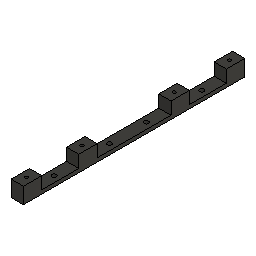
raspi_cover_holder (Autodesk Fusion 360 design; units mm, degrees)
Autodesk Fusion 360 part; units mm, degrees
sketch "Skizze1" plane through (0, 0, 0) normal (0, 0, 1) x (1, 0, 0)
  line L0 (0, 118.8766) -> (0, -120.4869) construction
  line L1 (5, -90) -> (-5, -90)
  line L2 (-5, -90) -> (-5, 90)
  line L3 (-5, 90) -> (5, 90)
  line L4 (5, 90) -> (5, -90)
  line L5 (5, -90) -> (-5, 90) construction
  line L6 (-5, -90) -> (5, 90) construction
  circle A0 centre (0, 37.5) radius 1.25
  circle A1 centre (0, -37.5) radius 1.25
  circle A2 centre (0, 15) radius 1.75
  circle A3 centre (0, -15) radius 1.75
  circle A4 centre (0, 60) radius 1.75
  circle A5 centre (0, -60) radius 1.75
  line L7 (-5, 30) -> (5, 30)
  line L8 (-5, -30) -> (5, -30)
  line L9 (-5, -45) -> (5, -45)
  line L10 (-5, 45) -> (5, 45)
  line L11 (1.2702, -39.7) -> (2.5403, -37.5)
  line L12 (2.5403, -37.5) -> (1.2702, -35.3)
  line L13 (1.2702, -35.3) -> (-1.2702, -35.3)
  line L14 (-1.2702, -35.3) -> (-2.5403, -37.5)
  line L15 (-2.5403, -37.5) -> (-1.2702, -39.7)
  line L16 (-1.2702, -39.7) -> (1.2702, -39.7)
  line L17 (1.2702, 35.3) -> (2.5403, 37.5)
  line L18 (2.5403, 37.5) -> (1.2702, 39.7)
  line L19 (1.2702, 39.7) -> (-1.2702, 39.7)
  line L20 (-1.2702, 39.7) -> (-2.5403, 37.5)
  line L21 (-2.5403, 37.5) -> (-1.2702, 35.3)
  line L22 (-1.2702, 35.3) -> (1.2702, 35.3)
  circle A6 centre (0, 82.5) radius 1.25
  circle A7 centre (0, -82.5) radius 1.25
  line L23 (1.2702, 80.3) -> (2.5403, 82.5)
  line L24 (2.5403, 82.5) -> (1.2702, 84.7)
  line L25 (1.2702, 84.7) -> (-1.2702, 84.7)
  line L26 (-1.2702, 84.7) -> (-2.5403, 82.5)
  line L27 (-2.5403, 82.5) -> (-1.2702, 80.3)
  line L28 (-1.2702, 80.3) -> (1.2702, 80.3)
  line L29 (1.2702, -84.7) -> (2.5403, -82.5)
  line L30 (2.5403, -82.5) -> (1.2702, -80.3)
  line L31 (1.2702, -80.3) -> (-1.2702, -80.3)
  line L32 (-1.2702, -80.3) -> (-2.5403, -82.5)
  line L33 (-2.5403, -82.5) -> (-1.2702, -84.7)
  line L34 (-1.2702, -84.7) -> (1.2702, -84.7)
  line L35 (-5, -75) -> (5, -75)
  line L36 (-5, 75) -> (5, 75)
  point P0 (0, -37.5)
  point P1 (0, 37.5)
  point P2 (0, 82.5)
  point P3 (0, -82.5)
  dimension "d1" = 10
  dimension "d2" = 180
  dimension "d3" = 37.5
  dimension "d4" = 37.5
  dimension "d5" = 2.5
  dimension "d7" = 2.5
  dimension "d8" = 3.5
  dimension "d9" = 3.5
  dimension "d10" = 15
  dimension "d11" = 15
  dimension "d12" = 3.5
  dimension "d13" = 3.5
  dimension "d14" = 45
  dimension "d15" = 45
  dimension "d16" = 7.5
  dimension "d17" = 7.5
  dimension "d20" = 4.4
  dimension "d21" = 4.4
  dimension "d33" = 2.5
  dimension "d34" = 2.5
  dimension "d35" = 4.4
  dimension "d36" = 4.4
  dimension "d37" = 45
  dimension "d38" = 45
  dimension "d39" = 7.5
  dimension "d40" = 7.5
  dimension "d41" = 7.5
  dimension "d42" = 7.5
  dimension "d43" = 7.5
  constraint vertical L0
  constraint coincident origin L0
  constraint horizontal L1
  constraint perpendicular L1 L2
  constraint parallel L1 L3
  constraint parallel L2 L4
  constraint coincident L5 origin
  constraint coincident L6 origin
  constraint coincident L0 P1
  constraint coincident L0 P0
  constraint coincident L0 A2.centre
  constraint coincident L0 A3.centre
  constraint coincident L0 A4.centre
  constraint coincident L0 A5.centre
  constraint coincident L2 L7.start
  constraint coincident L4 L7.end
  constraint perpendicular L4 L7
  constraint coincident L2 L8.start
  constraint coincident L4 L8.end
  constraint perpendicular L4 L8
  constraint coincident L2 L9.start
  constraint coincident L4 L9.end
  constraint perpendicular L4 L9
  constraint coincident L2 L10.start
  constraint coincident L4 L10.end
  constraint perpendicular L4 L10
  constraint coincident P0 A1.centre
  constraint coincident P1 A0.centre
  constraint horizontal L22
  constraint horizontal L16
  constraint coincident L0 P2
  constraint coincident L0 P3
  constraint coincident P2 A6.centre
  constraint coincident P3 A7.centre
  constraint horizontal L34
  constraint horizontal L28
  constraint coincident L2 L35.start
  constraint coincident L4 L35.end
  constraint perpendicular L4 L35
  constraint coincident L2 L36.start
  constraint coincident L4 L36.end
  constraint perpendicular L4 L36
  measures "d1" distance of L2 L4
  measures "d2" distance of L1 L3
  measures "d3" distance of origin A1.centre
  measures "d4" distance of origin P1
  measures "d5" diameter of A0
  measures "d7" diameter of A1
  measures "d8" diameter of A3
  measures "d9" diameter of A2
  measures "d10" distance of origin A2.centre
  measures "d11" distance of origin A3.centre
  measures "d12" diameter of A5
  measures "d13" diameter of A4
  measures "d14" distance of A2.centre A4.centre
  measures "d15" distance of A3.centre A5.centre
  measures "d16" distance of P0 L9
  measures "d17" distance of P1 L10
  measures "d20" distance of L13 L16
  measures "d21" distance of L19 L22
  measures "d33" diameter of A7
  measures "d34" diameter of A6
  measures "d35" distance of L25 L28
  measures "d36" distance of L31 L34
  measures "d37" distance of P0 P3
  measures "d38" distance of P1 P2
  measures "d39" distance of P0 L8
  measures "d40" distance of L1 P3
  measures "d41" distance of P3 L35
  measures "d42" distance of P1 L7
  measures "d43" distance of P2 L36
extrude "Extrusion1" add sketch "Skizze1" along normal blind 3 contours L1 L2 L4 L35 | L2 L4 L9 L35 | L2 L4 L8 L9 | L2 L4 L7 L8 | L2 L4 L7 L10 | L2 L4 L10 L36 | L2 L3 L4 L36 | L11 L12 L13 L14 L15 L16 | L17 L18 L19 L20 L21 L22 | L23 L24 L25 L26 L27 L28 | L29 L30 L31 L32 L33 L34
extrude "Extrusion2" add sketch "Skizze1" along normal blind 13 contours L1 L2 L4 L35 | L2 L4 L8 L9 | L2 L4 L7 L10 | L2 L3 L4 L36 | L11 L12 L13 L14 L15 L16 | L17 L18 L19 L20 L21 L22 | L23 L24 L25 L26 L27 L28 | L29 L30 L31 L32 L33 L34
extrude "Extrusion3" cut sketch "Skizze1" along normal blind 11 contours L11 L12 L13 L14 L15 L16 | L17 L18 L19 L20 L21 L22 | L23 L24 L25 L26 L27 L28 | L29 L30 L31 L32 L33 L34
extrude "Extrusion4" add sketch "Skizze1" along normal blind 9.2 contours L11 L12 L13 L14 L15 L16 | L17 L18 L19 L20 L21 L22 | L23 L24 L25 L26 L27 L28 | L29 L30 L31 L32 L33 L34
equation "d3 = ( 75 / 2 ) * 1 mm"
equation "d4 = ( 75 / 2 ) * 1 mm"
named bodies: "raspi_cover_holder"
